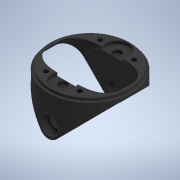
# Autodesk Inventor part: SingleBracket
Saved by Autodesk Inventor 2020 (Build 240168000, 168)
## iProperties
Created: 2019-05-27
Part Number: SingleBracket
Material: ABS Plastic
Document SubType Name: Modeling
Designer: Connor
Density: 1.06 g/cm^3
Appearance: Rubber - Black
Author: Connor
Autodesk Inventor part; units mm, degrees
sketch "Sketch1" plane through (0, 0, 0) normal (0, 0, 1) x (1, 0, 0)
  circle A0 centre (0, 0) radius 50.8 construction
  circle A1 centre (0, 0) radius 53.975 construction
  circle A2 centre (0, 0) radius 6.35
  circle A3 centre (0, 0) radius 12.7
  line L0 (0, 31.75) -> (46.99, 31.75)
  line L1 (46.99, 31.75) -> (46.99, -12.7)
  line L2 (46.99, -12.7) -> (0, -12.7)
  line L3 (0, -12.7) -> (0, 31.75)
  line L4 (9.0201, -8.9402) -> (46.99, 29.3687)
  line L5 (0, 31.75) -> (44.45, 31.75)
  line L6 (44.45, 31.75) -> (44.45, 34.925)
  line L7 (44.45, 34.925) -> (0, 34.925)
  line L8 (0, 34.925) -> (0, 31.75)
  point P0 (0, -12.7)
  dimension "d3" = 25.4
  dimension "d0" = 101.6
  dimension "d1" = 3.175
  dimension "d2" = 12.7
  dimension "d5" = 31.75
  dimension "d7" = 2.3813
  dimension "d15" = 44.45
  dimension "d16" = 2.54
  dimension "d17" = 3.175
  constraints: 18 end point, 4 parallel, 3 centre point, 3 coincident, 3 horizontal, 2 perpendicular, 2 point on line, 4 other
  measures "d0" diameter of A0
  measures "d1" radial gap between concentric circles of A0 A1
  measures "d2" diameter of A2
  measures "d5" distance from line of point (0, 0) L0
  measures "d7" distance from line of L0 L4.end
  measures "d15" distance of L6.end L7.end
  measures "d16" distance between parallel lines of L6 L1
  measures "d17" distance between parallel lines of L5 L7
revolve "Revolution1" add sketch "Sketch1" angle 360 about axis through (0, -12.7, 0) along (0, 1, 0) picked at (2.0636, 0.471) picked at (10.4241, 1.413) contours A2 L3 | A2 L3 A3 | L3 L0 L1 L4 A3 | A3 L4 L1 L2 | L8 L7 L6 L0
extrude "Extrusion1" cut sketch "Sketch1" along normal through all both and the other way through all contours A3 L4 L1 L2
mirror "Mirror1" about plane through (0, 0, 0) normal (1, 0, 0) of "Extrusion1"
sketch "Sketch5" plane through (0, 0, 0) normal (0, 1, 0) x (-1, 0, 0)
  line L0 (0, 0) -> (-53.975, 0)
  line L1 (-53.975, 0) -> (-53.975, -6.35)
  line L2 (-34.925, -25.4) -> (0, -25.4)
  line L3 (0, -25.4) -> (0, 0)
  line L4 (0, 0) -> (-53.975, 0)
  line L5 (-53.975, -6.35) -> (-53.975, 6.35)
  line L6 (-34.925, 25.4) -> (0, 25.4)
  line L7 (0, 25.4) -> (0, 0)
  arc A0 (-53.975, -6.35) -> (-34.925, -25.4) centre (-34.925, -6.35) ccw
  arc A1 (-34.925, 25.4) -> (-53.975, 6.35) centre (-34.925, 6.35) ccw
  point P0 (-53.975, -25.4)
  point P1 (-53.975, 25.4)
  dimension "d32" = 50.8
  dimension "d33" = 53.975
  dimension "d37" = 12.7
  constraints: 16 end point, 5 point on line, 4 parallel, 4 point on circle, 4 tangent, 2 centre point, 2 collinear, 2 horizontal, 2 perpendicular, 1 equal radius, 1 midpoint
  measures "d32" distance between parallel lines of L6 L2
  measures "d33" distance between parallel lines of L3 L1
  measures "d37" distance of L5.start L5.end
revolve "Revolution3" cut sketch "Sketch5" angle 360 about axis through (0, 0, -25.4) along (0, 0, 1)
ref_plane "Work Plane1" through (0, 9.525, 46.99) normal (0, 0, 1) x (1, 0, 0)
sketch "Sketch6" plane through (0, 9.525, 46.99) normal (0, 0, 1) x (1, 0, 0)
  point P0 (0, -9.525)
  point P1 (0, -9.525)
  constraints: 1 coincident
hole "Hole1" at (0, 0, 46.99) direction (0, 0, -1) diameter 12.7 depth 77.7875 counterbore diameter 19.05 counterbore depth 7.9375
sketch "Sketch7" plane through (0, 0, -30.7975) normal (0, 0, 1) x (1, 0, 0)
  circle A0 centre (0, 0) radius 4.7625
  dimension "d48" = 9.525
  constraints: 1 centre point, 1 coincident
  measures "d48" diameter of A0
extrude "Extrusion3" cut sketch "Sketch7" against normal blind 15.875
ref_plane "Work Plane3" through (0, 0, -40.3225) normal (0, 0, 1) x (1, 0, 0)
sketch "Sketch9" plane through (0, 0, -40.3225) normal (0, 0, 1) x (1, 0, 0)
  circle A0 centre (0, 0) radius 4.7625 projected
  line L0 (0, 8.2489) -> (7.1438, 4.1244)
  line L1 (7.1438, 4.1244) -> (7.1437, -4.1244)
  line L2 (7.1437, -4.1244) -> (0, -8.2489)
  line L3 (0, -8.2489) -> (-7.1438, -4.1244)
  line L4 (-7.1438, -4.1244) -> (-7.1437, 4.1244)
  line L5 (-7.1437, 4.1244) -> (0, 8.2489)
  dimension "d55" = 14.2875
  constraints: 12 end point, 1 coincident, 1 vertical alignment, 13 other
  measures "d55" distance between parallel lines of L3 L0
extrude "Extrusion5" cut sketch "Sketch9" along normal blind 6.35
ref_plane "Work Plane4" through (0, -12.7, 0) normal (0, 1, 0) x (-1, 0, 0)
sketch "Sketch11" plane through (0, -12.7, 0) normal (0, 1, 0) x (-1, 0, 0)
  line L0 (-7.1437, -40.3225) -> (-7.1437, -33.9725) projected
  line L1 (7.1438, -40.3225) -> (7.1438, -33.9725) projected
  line L2 (7.1438, -40.3225) -> (0, -40.3225) projected
  line L3 (0, -40.3225) -> (-7.1437, -40.3225) projected
  line L4 (0, -33.9725) -> (-7.1437, -33.9725) projected
  line L5 (7.1438, -33.9725) -> (0, -33.9725) projected
  point P0 (0, 0)
extrude "Extrusion6" cut sketch "Sketch11" along normal up to surface (16.8244 mm away)
sketch "Sketch12" plane through (0, 34.925, 0) normal (0, 1, 0) x (1, 0, 0)
  circle A0 centre (0, -30.48) radius 12.7
  circle A1 centre (0, 30.48) radius 12.7
  line L0 (0, -30.48) -> (0, 0) construction
  line L1 (0, 0) -> (0, 30.48) construction
  dimension "d64" = 60.96
  dimension "d65" = 25.4
  constraints: 4 end point, 2 centre point, 2 collinear, 1 equal radius, 1 vertical
  measures "d64" distance of L1.end L0.start
  measures "d65" diameter of A0
extrude "Extrusion7" cut sketch "Sketch12" against normal blind 3.175
sketch "Sketch14" plane through (0, -12.7, 0) normal (0, 1, 0) x (-1, 0, 0)
  line L0 (-19.05, 30.48) -> (19.05, 30.48) construction
  line L1 (19.05, 30.48) -> (19.05, -30.48) construction
  line L2 (19.05, -30.48) -> (-19.05, -30.48) construction
  line L3 (-19.05, -30.48) -> (-19.05, 30.48) construction
  line L4 (-19.05, 30.48) -> (19.05, -30.48) construction
  line L5 (19.05, 30.48) -> (-19.05, -30.48) construction
  point P0 (0, 0)
  point P1 (0, 0)
  dimension "d68" = 60.96
  dimension "d69" = 38.1
  constraints: 12 end point, 5 coincident, 2 parallel, 1 horizontal, 1 midpoint, 1 perpendicular
  measures "d68" distance of L2.end L0.start
  measures "d69" distance between parallel lines of L1 L3
hole "Hole2" at (19.05, -12.7, 30.48) at (19.05, -12.7, -30.48) at (-19.05, -12.7, -30.48) at (-19.05, -12.7, 30.48) direction (0, 1, 0) diameter 5.1594 end through all counterbore diameter 7.9375 counterbore depth 22.225
fillet "Fillet15" radius 0.7937 10 edges at (-19.05, 1.1792, -26.5112) (-19.05, 1.1792, 34.4488) (19.05, 1.1792, 34.4488) (19.05, 1.1792, -26.5112) (9.525, -0.0106, 46.0145) (-9.525, -0.0115, 46.0145) (0, -12.7, -33.9725) (0, -12.7, -40.3225) (7.1437, -10.5003, -37.1475) (-7.1438, -10.5003, -37.1475)
sketch "Sketch15" plane through (0, 31.75, 0) normal (0, 1, 0) x (1, 0, 0)
  arc A0 (-11.5989, -25.3074) -> (11.5989, -25.3074) centre (0, -30.48) ccw projected
  circle A1 centre (0, -30.48) radius 4.7625
  circle A2 centre (0, 30.48) radius 4.7625
  arc A3 (11.5989, 25.3074) -> (-11.5989, 25.3074) centre (0, 30.48) ccw projected
  point P0 (0, 0)
  dimension "d79" = 9.525
  constraints: 2 centre point, 1 coincident, 1 concentric, 1 equal radius
  measures "d79" diameter of A1
extrude "Extrusion8" cut sketch "Sketch15" against normal blind 3.175
body "Solid1"
